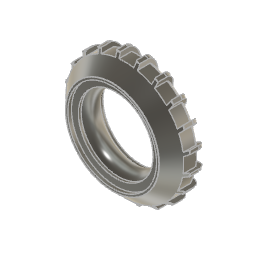
beeboy (Autodesk Fusion 360 archive; units mm, degrees)
design "tire"
Autodesk Fusion 360 part; units mm, degrees
sketch "Sketch1" plane through (0, 0, 0) normal (1, 0, 0) x (0, 1, 0)
  line L0 (0, 18.646) -> (0, 0) construction
  line L1 (-2.038, 12.646) -> (0, 12.646)
  arc A0 (-2.038, 12.646) -> (-3.3919, 11.016) centre (0, 9.5759) ccw
  line L2 (-3.3919, 11.016) -> (-3.3919, 9.516)
  line L3 (-3.3919, 9.516) -> (-2.6249, 9.516)
  line L4 (-2.6249, 9.516) -> (-2.6249, 8.016)
  line L5 (-2.6249, 8.016) -> (-2.0439, 8.016)
  arc A1 (-2.0439, 8.016) -> (0, 6.8505) centre (0, 9.2255) ccw
  line L6 (2.038, 12.646) -> (0, 12.646)
  arc A2 (3.3919, 11.016) -> (2.038, 12.646) centre (0, 9.5759) ccw
  line L7 (3.3919, 11.016) -> (3.3919, 9.516)
  line L8 (3.3919, 9.516) -> (2.6249, 9.516)
  line L9 (2.6249, 9.516) -> (2.6249, 8.016)
  line L10 (2.6249, 8.016) -> (2.0439, 8.016)
  arc A3 (0, 6.8505) -> (2.0439, 8.016) centre (0, 9.2255) ccw
  dimension "d22" = 12.646
  dimension "d23" = 2.038
  dimension "d25" = 3.685
  dimension "d26" = 0.767
  dimension "d27" = 1.5
  dimension "d28" = 1.5
  dimension "d29" = 0.581
  dimension "d32" = 2.375
  dimension "d34" = 2.634
  dimension "d35" = 3.13
  dimension "d36" = 3.3919
  constraint coincident L0.end origin
  constraint vertical L0
  constraint coincident L0 L1.end
  constraint perpendicular L0 L1
  constraint coincident L0 A0.centre
  constraint vertical L2
  constraint perpendicular L2 L3
  constraint perpendicular L3 L4
  constraint perpendicular L4 L5
  constraint coincident L0 A1.centre
  constraint coincident L0 A1.end
  constraint symmetric L0 L1.start L6.start
  constraint symmetric L0 L1.end L6.end
  constraint symmetric L0 A0.end A2.start
  constraint symmetric L0 A0 A2
  constraint symmetric L0 L2.end L7.end
  constraint symmetric L0 L3.end L8.end
  constraint symmetric L0 L4.end L9.end
  constraint symmetric L0 L5.end L10.end
  constraint symmetric L0 A1.end A3.start
  constraint symmetric L0 A1 A3
  measures "d22" vertical distance of L0.end L1.start
  measures "d23" distance of L1.start L1.end
  measures "d25" radius of A0
  measures "d26" distance of L2.end L3.end
  measures "d27" distance of L3.end L4.end
  measures "d28" distance of A0.end L2.end
  measures "d29" distance of L4.end L5.end
  measures "d32" radius of A1
  measures "d35" distance of L1 L3
  measures "d36" distance of L0 L2
sketch "Sketch2" plane through (0, 0, 0) normal (1, 0, 0) x (0, 1, 0)
revolve "Revolve1" add sketch "Sketch1" angle 360 about axis through (0, 1.75, 0) along (0, 1, 0)
sketch "Sketch3" plane through (0, -3.3919, 0) normal (0, -1, 0) x (1, 0, 0)
  circle A0 centre (0, 0) radius 9.516
  circle A1 centre (0, 0) radius 11.016
  line L0 (-0.3, 0) -> (-0.3, 9.5113) construction
  line L1 (-0.3, 9.5113) -> (0.5, 9.5113)
  line L2 (0.5, 9.5113) -> (-1.6939, 13.3113)
  line L3 (-1.6939, 13.3113) -> (-2.4939, 13.3113)
  line L4 (-2.4939, 13.3113) -> (-0.3, 9.5113)
  dimension "d38" = 0.3
  dimension "d39" = 3.8
  dimension "d40" = 120
  dimension "d41" = 0.8
  dimension "d42" = 0.8
  constraint vertical L0
  constraint coincident A0 L0.end
  constraint perpendicular L0 L1
  constraint parallel L1 L3
  measures "d38" distance of L0.start A0.centre
  measures "d39" vertical distance of L0.end L3.end
  measures "d40" angle of L1 L4
  measures "d41" distance of L0.end L1.end
  measures "d42" distance of L2.end L3.end
extrude "Extrude1" add sketch "Sketch3" against normal blind 6.784 contours A1 L1 L2 L4 | A1 L2 L3 L4 picked at (-0.0551, 10.0108)
fillet "Fillet1" radius 1.5 2 edges at (-2.0939, 3.3921, 13.3113) (-2.0939, -3.3919, 13.3113)
pattern_circular "C-Pattern1" count 20 over 360 about axis through (0, 0, 0) along (0, 1, 0) of "Extrude1", "Fillet1"
sketch "Sketch4" plane through (0, 0, 0) normal (1, 0, 0) x (0, 1, 0)
  line L0 (-3.4722, 10.016) -> (-3.2952, 10.016)
  line L1 (-3.2952, 10.016) -> (0.0001, 13.3113)
  line L2 (0.0001, 13.3113) -> (-4.457, 13.3113)
  line L3 (-4.457, 13.3113) -> (-4.457, 10.016)
  line L4 (-4.457, 10.016) -> (-3.4722, 10.016)
  line L5 (-1.8919, 13.3113) -> (1.8921, 13.3113)
  line L6 (-4.457, 13.3113) -> (-4.457, 15)
  line L7 (-4.457, 15) -> (0, 15)
  line L8 (0, 15) -> (0.0001, 13.3113)
  point P0 (-3.3919, 9.516)
  point P1 (-3.3919, 11.0099)
  dimension "d49" = 0.5
  dimension "d50" = 0.177
  dimension "d51" = 135
  dimension "d52" = 45
  constraint horizontal L0
  constraint parallel L0 L2
  constraint perpendicular L2 L3
  constraint perpendicular L3 L4
  constraint midpoint L1.end L5
  constraint perpendicular L2 L6
  constraint perpendicular L3 L7
  measures "d49" distance of P0 L4
  measures "d50" distance of L0.start L0.end
  measures "d51" angle of L0 L1
  measures "d52" angle of L1 L5
revolve "Revolve2" cut sketch "Sketch4" angle 360 about axis through (0, 1.75, 0) along (0, 1, 0)
